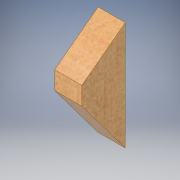
# Autodesk Inventor part: feet
Saved by Autodesk Inventor 2019 (Build 230136000, 136)
## iProperties
Created: 2019-05-05
Part Number: feet
Material: Madeira
Document SubType Name: Modeling
Designer: Daniel Regner
Density: 0.570257 g/cm^3
Appearance: Pinho amarelo - Sólido natural sem brilho
lenght: 25,000 mm
widht: 40,000 mm
Author: Daniel Regner
Autodesk Inventor part; units mm, degrees
ref_plane "YZ Plane" through (0, 0, 0) normal (1, 0, 0) x (0, 1, 0)
ref_plane "XZ Plane" through (0, 0, 0) normal (0, 1, 0) x (-1, 0, 0)
ref_plane "XY Plane" through (0, 0, 0) normal (0, 0, 1) x (1, 0, 0)
sketch "Esboço1" plane through (0, 0, 0) normal (0, 1, 0) x (-1, 0, 0)
  line L0 (-12.5, 20) -> (12.5, 20)
  line L1 (12.5, 20) -> (12.5, -20)
  line L2 (12.5, -20) -> (-12.5, -20)
  line L3 (-12.5, -20) -> (-12.5, 20)
  line L4 (-12.5, 20) -> (12.5, -20) construction
  line L5 (12.5, 20) -> (-12.5, -20) construction
  point P0 (0, 0)
  dimension "lenght" = 25
  dimension "widht" = 40
  constraints: 12 end point, 2 midpoint, 2 parallel, 1 horizontal, 1 perpendicular
  measures "lenght" distance of L1.end L2.end
  measures "widht" distance of L0.end L1.end
extrude "Extrusão1" add sketch "Esboço1" along normal mid plane 100
sketch "Esboço2" plane through (12.5, -50, -20) normal (1, 0, 0) x (0, 0, -1)
  line L0 (0, 100) -> (0, 0) projected
  line L1 (0, 100) -> (-40, 70)
  line L2 (-40, 0) -> (-40, 100) projected
  line L3 (-40, 70) -> (-40, 100)
  line L4 (-40, 100) -> (0, 100)
  point P0 (-20, 50)
  dimension "d4" = 50
  constraints: 6 end point, 1 collinear, 1 perpendicular, 1 point on line
  measures "d4" distance of L0.start L1.end
extrude "Extrusão2" cut sketch "Esboço2" against normal blind 25
sketch "Esboço3" plane through (12.5, -50, 20) normal (1, 0, 0) x (0, 0, -1)
  line L0 (0, 0) -> (40, 0) projected
  line L1 (40, 0) -> (0, 53.3331)
  line L2 (0, 70) -> (0, 0) projected
  line L3 (0, 53.3331) -> (0, 0)
  line L4 (0, 0) -> (40, 0)
  point P0 (20, 50)
  dimension "d7" = 36.87
  constraints: 6 end point, 1 collinear, 1 perpendicular, 1 point on line
  measures "d7" angle of L2 L1
extrude "Extrusão3" cut sketch "Esboço3" against normal blind 25
equation "\"lenght\" = RIP_L"
equation "\"widht\" = RIP_H"
equation "\"d5\" = RIP_L"
equation "\"d8\" = RIP_L"
equation "\"RIP_H\" = 40"
equation "\"RIP_L\" = 25"
